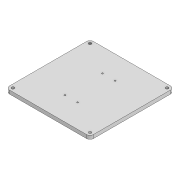
# Autodesk Inventor part: Arena
Saved by Autodesk Inventor 2020 (Build 240168000, 168)
## iProperties
Created: 2020-08-28
Part Number: Arena
Material: Generic
Document SubType Name: Modeling
Designer: ferrerx
Density: 1 g/cm^3
Appearance: Default
Author: ferrerx
Autodesk Inventor part; units mm, degrees
ref_plane "YZ Plane" through (0, 0, 0) normal (1, 0, 0) x (0, 1, 0)
ref_plane "XZ Plane" through (0, 0, 0) normal (0, 1, 0) x (-1, 0, 0)
ref_plane "XY Plane" through (0, 0, 0) normal (0, 0, 1) x (1, 0, 0)
sketch "Sketch1" plane through (0, 0, 0) normal (0, 1, 0) x (-1, 0, 0)
  line L0 (-60, 60) -> (60, 60)
  line L1 (60, 60) -> (60, -60)
  line L2 (60, -60) -> (-60, -60)
  line L3 (-60, -60) -> (-60, 60)
  line L4 (-60, 60) -> (60, -60) construction
  line L5 (60, 60) -> (-60, -60) construction
  point P0 (0, 0)
  dimension "d0" = 120
  dimension "d1" = 120
  constraints: 12 end point, 2 midpoint, 2 parallel, 1 horizontal, 1 perpendicular
  measures "d0" distance of L1.end L2.end
  measures "d1" distance of L0.end L1.end
extrude "Extrusion1" add sketch "Sketch1" along normal blind 5
sketch "Sketch2" plane through (0, 5, 0) normal (0, 1, 0) x (1, 0, 0)
  line L0 (55, -55) -> (-55, -55) construction
  line L1 (-55, -55) -> (-55, 55) construction
  line L2 (-55, 55) -> (55, 55) construction
  line L3 (55, 55) -> (55, -55) construction
  line L4 (55, -55) -> (-55, 55) construction
  line L5 (-55, -55) -> (55, 55) construction
  circle A0 centre (-55, 55) radius 2
  circle A1 centre (-55, -55) radius 2
  circle A2 centre (55, 55) radius 2
  circle A3 centre (55, -55) radius 2
  point P0 (0, 0)
  dimension "d4" = 110
  dimension "d5" = 110
  dimension "d6" = 4
  dimension "d7" = 4
  dimension "d8" = 4
  dimension "d9" = 4
  constraints: 12 end point, 4 centre point, 4 coincident, 2 midpoint, 2 parallel, 1 horizontal, 1 perpendicular
  measures "d4" distance of L1.end L2.end
  measures "d5" distance of L2.end L0.start
  measures "d6" diameter of A0
  measures "d7" diameter of A3
  measures "d8" diameter of A2
  measures "d9" diameter of A1
extrude "Extrusion2" cut sketch "Sketch2" against normal blind 5
fillet "Fillet1" radius 5 4 edges at (60, 2.5, -60) (60, 2.5, 60) (-60, 2.5, -60) (-60, 2.5, 60)
sketch "Sketch3" plane through (0, 5, 0) normal (0, 1, 0) x (1, 0, 0)
  line L0 (-35.5, -35.5) -> (35.5, -35.5) construction
  line L1 (35.5, -35.5) -> (35.5, 35.5) construction
  line L2 (35.5, 35.5) -> (-35.5, 35.5) construction
  line L3 (-35.5, 35.5) -> (-35.5, -35.5) construction
  line L4 (-35.5, -35.5) -> (35.5, 35.5) construction
  line L5 (35.5, -35.5) -> (-35.5, 35.5) construction
  circle A0 centre (9, 26.8) radius 1
  circle A1 centre (-9, 26.8) radius 1
  circle A2 centre (-9, -26.8) radius 1
  circle A3 centre (9, -26.8) radius 1
  point P0 (0, 0)
  dimension "d13" = 71
  dimension "d14" = 71
  dimension "d15" = 26.5
  dimension "d16" = 8.7
  dimension "d17" = 2
  dimension "d18" = 8.7
  dimension "d19" = 2
  dimension "d20" = 26.5
  dimension "d21" = 26.5
  dimension "d22" = 26.5
  dimension "d23" = 8.7
  dimension "d24" = 2
  dimension "d25" = 8.7
  dimension "d26" = 2
  constraints: 12 end point, 4 centre point, 2 midpoint, 2 parallel, 1 horizontal, 1 perpendicular
  measures "d13" distance of L0.end L1.end
  measures "d14" distance of L0.start L0.end
  measures "d15" distance from line of L1 A0.centre
  measures "d16" distance from line of L2 A0.centre
  measures "d17" diameter of A0
  measures "d18" distance from line of L2 A1.centre
  measures "d19" diameter of A1
  measures "d20" distance from line of L3 A1.centre
  measures "d21" distance from line of L1 A3.centre
  measures "d22" distance from line of L3 A2.centre
  measures "d23" distance from line of L0 A2.centre
  measures "d24" diameter of A2
  measures "d25" distance from line of L0 A3.centre
  measures "d26" diameter of A3
extrude "Extrusion3" cut sketch "Sketch3" against normal blind 10
body "Solid1"
